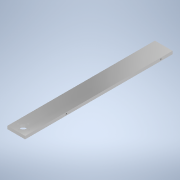
# Autodesk Inventor part: 横長3rdフラットバー
Saved by Autodesk Inventor 2022 (Build 260153000, 153)
## iProperties
Created: 2022-11-07
Part Number: 横長3rdフラットバー
Material: アルミニウム 6061
Document SubType Name: Modeling
Designer: tdn82
Density: 2.7 g/cm^3
Appearance: アルミニウム - フラット
Author: tdn82
Autodesk Inventor part; units mm, degrees
ref_plane "YZ Plane" through (0, 0, 0) normal (1, 0, 0) x (0, 1, 0)
ref_plane "XZ Plane" through (0, 0, 0) normal (0, 1, 0) x (-1, 0, 0)
ref_plane "XY Plane" through (0, 0, 0) normal (0, 0, 1) x (1, 0, 0)
sketch "スケッチ1" plane through (0, 0, 0) normal (0, 1, 0) x (-1, 0, 0)
  line L0 (0, 0) -> (-30, 0)
  line L1 (-30, 0) -> (-30, -250)
  line L2 (-30, -250) -> (0, -250)
  line L3 (0, -250) -> (0, 0)
  point P0 (-15, -12)
  dimension "d0" = 250
  dimension "d1" = 30
  dimension "d4" = 15
  dimension "d5" = 12
  constraints: 8 end point, 2 parallel, 1 horizontal, 1 perpendicular
  measures "d0" distance of L2.end L0.start
  measures "d1" distance of L0.start L0.end
  measures "d4" distance from line of L3 point (-15, -12)
  measures "d5" distance from line of point (-15, -12) L0
extrude "押し出し1" add sketch "スケッチ1" along normal blind 5
sketch "スケッチ2" plane through (0, 0, 0) normal (0, -1, 0) x (1, 0, 0)
  line L0 (0, -250) -> (0, 0) projected
  line L1 (0, 0) -> (30, 0) projected
  point P0 (15, -12)
  dimension "d6" = 15
  dimension "d7" = 12
  measures "d6" distance from line of L0 point (15, -12)
  measures "d7" distance from line of point (15, -12) L1
hole "穴1" at (15, 0, -12) direction (0, 1, 0) diameter 11 end through all
sketch "スケッチ3" plane through (0, 0, 0) normal (0, -1, 0) x (1, 0, 0)
  line L0 (0, 0) -> (30, 0)
  circle A0 centre (15, -12) radius 4
  point P0 (23.5, -12)
  point P1 (15, -3.5)
  point P2 (6.5, -12)
  point P3 (15, -20.5)
  dimension "d17" = 360
  constraints: 2 end point, 1 centre point, 5 other
hole "穴2" at (23.5, 0, -12) at (15, 0, -3.5) at (6.5, 0, -12) at (15, 0, -20.5) direction (0, 1, 0) diameter 3 end through all
sketch "スケッチ4" plane through (0, 0, -250) normal (-1, 0, 0) x (0, 0, 1)
  line L0 (0, 5) -> (250, 5) projected
  line L1 (0, 0) -> (0, 5) projected
  point P0 (250, 0)
  point P1 (180, 2.5)
  point P2 (20, 2.5)
  dimension "d25" = 2.5
  dimension "d26" = 180
  dimension "d27" = 20
  measures "d25" distance from line of L0 point (180, 2.5)
  measures "d26" distance from line of L1 point (180, 2.5)
  measures "d27" distance from line of L1 point (20, 2.5)
hole "穴3" at (0, 2.5, -70) at (0, 2.5, -230) direction (1, 0, 0) diameter 2.459 end through all thread size "M3x0.5" class "6H" standard "ANSI Metric M Profile"
